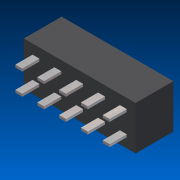
# Autodesk Inventor part: MOLEX
Saved by Autodesk Inventor 2015 SP1 (Build 190203100, 203)
## iProperties
Created: 2015-12-01
Part Number: MOLEX
Material: Generic
Document SubType Name: Modeling
Designer: User
Density: 1 g/cm^3
Appearance: Default
Author: User
Autodesk Inventor part; units mm, degrees
ref_plane "YZ Plane" through (0, 0, 0) normal (1, 0, 0) x (0, 1, 0)
ref_plane "XZ Plane" through (0, 0, 0) normal (0, 1, 0) x (-1, 0, 0)
ref_plane "XY Plane" through (0, 0, 0) normal (0, 0, 1) x (1, 0, 0)
sketch "Эскиз1" plane through (0, 0, 0) normal (0, 1, 0) x (-1, 0, 0)
  line L0 (6.5, -2.54) -> (-6.5, -2.54)
  line L1 (-6.5, -2.54) -> (-6.5, 2.54)
  line L2 (-6.5, 2.54) -> (6.5, 2.54)
  line L3 (6.5, 2.54) -> (6.5, -2.54)
  line L4 (0, -3.556) -> (0, 3.556) projected
  line L5 (9.1, 0) -> (-9.1, 0) projected
  point P0 (0, 0)
  dimension "d0" = 13
  dimension "d1" = 5.08
  constraints: 8 end point, 2 parallel, 1 horizontal, 1 perpendicular, 2 other
  measures "d0" distance of L1.end L2.end
  measures "d1" distance of L0.end L1.end
extrude "Выдавливание1" add sketch "Эскиз1" along normal blind 4.4
sketch "Эскиз2" plane through (0, 4.4, 0) normal (0, 1, 0) x (1, 0, 0)
  line L0 (-5.48, 1.67) -> (-4.68, 1.67)
  line L1 (-4.68, 1.67) -> (-4.68, 0.87)
  line L2 (-4.68, 0.87) -> (-5.48, 0.87)
  line L3 (-5.48, 0.87) -> (-5.48, 1.67)
  line L4 (-2.94, 1.67) -> (-2.14, 1.67)
  line L5 (-2.14, 1.67) -> (-2.14, 0.87)
  line L6 (-2.14, 0.87) -> (-2.94, 0.87)
  line L7 (-2.94, 0.87) -> (-2.94, 1.67)
  line L8 (-0.4, 1.67) -> (0.4, 1.67)
  line L9 (0.4, 1.67) -> (0.4, 0.87)
  line L10 (0.4, 0.87) -> (-0.4, 0.87)
  line L11 (-0.4, 0.87) -> (-0.4, 1.67)
  line L12 (2.14, 1.67) -> (2.94, 1.67)
  line L13 (2.94, 1.67) -> (2.94, 0.87)
  line L14 (2.94, 0.87) -> (2.14, 0.87)
  line L15 (2.14, 0.87) -> (2.14, 1.67)
  line L16 (4.68, 1.67) -> (5.48, 1.67)
  line L17 (5.48, 1.67) -> (5.48, 0.87)
  line L18 (5.48, 0.87) -> (4.68, 0.87)
  line L19 (4.68, 0.87) -> (4.68, 1.67)
  line L20 (-5.48, -0.87) -> (-4.68, -0.87)
  line L21 (-4.68, -0.87) -> (-4.68, -1.67)
  line L22 (-4.68, -1.67) -> (-5.48, -1.67)
  line L23 (-5.48, -1.67) -> (-5.48, -0.87)
  line L24 (-2.94, -0.87) -> (-2.14, -0.87)
  line L25 (-2.14, -0.87) -> (-2.14, -1.67)
  line L26 (-2.14, -1.67) -> (-2.94, -1.67)
  line L27 (-2.94, -1.67) -> (-2.94, -0.87)
  line L28 (-0.4, -0.87) -> (0.4, -0.87)
  line L29 (0.4, -0.87) -> (0.4, -1.67)
  line L30 (0.4, -1.67) -> (-0.4, -1.67)
  line L31 (-0.4, -1.67) -> (-0.4, -0.87)
  line L32 (2.14, -0.87) -> (2.94, -0.87)
  line L33 (2.94, -0.87) -> (2.94, -1.67)
  line L34 (2.94, -1.67) -> (2.14, -1.67)
  line L35 (2.14, -1.67) -> (2.14, -0.87)
  line L36 (4.68, -0.87) -> (5.48, -0.87)
  line L37 (5.48, -0.87) -> (5.48, -1.67)
  line L38 (5.48, -1.67) -> (4.68, -1.67)
  line L39 (4.68, -1.67) -> (4.68, -0.87)
  line L40 (0, 3.556) -> (0, -3.556) projected
  line L41 (-9.1, 0) -> (9.1, 0) projected
  point P0 (0, 0)
  dimension "d4" = 0.8
  dimension "d5" = 0.8
  dimension "d8" = 2.54
  dimension "d11" = 2.54
  constraints: 80 end point, 2 collinear, 2 horizontal, 2 parallel, 1 perpendicular, 1 vertical, 72 other
  measures "d4" distance of L1.end L2.end
  measures "d5" distance of L0.end L1.end
  measures "d8" distance of L0.start L4.start
  measures "d11" distance of L0.start L20.start
extrude "Выдавливание2" cut sketch "Эскиз2" against normal blind 4
sketch "Эскиз3" plane through (0, 0, 0) normal (0, -1, 0) x (1, 0, 0)
  line L0 (0, -3.556) -> (0, 3.556) projected
  line L1 (-9.1, 0) -> (9.1, 0) projected
  line L2 (-5.48, 1.42) -> (-4.68, 1.42)
  line L3 (-4.68, 1.42) -> (-4.68, 1.12)
  line L4 (-4.68, 1.12) -> (-5.48, 1.12)
  line L5 (-5.48, 1.12) -> (-5.48, 1.42)
  line L6 (-2.94, 1.42) -> (-2.14, 1.42)
  line L7 (-2.14, 1.42) -> (-2.14, 1.12)
  line L8 (-2.14, 1.12) -> (-2.94, 1.12)
  line L9 (-2.94, 1.12) -> (-2.94, 1.42)
  line L10 (-0.4, 1.42) -> (0.4, 1.42)
  line L11 (0.4, 1.42) -> (0.4, 1.12)
  line L12 (0.4, 1.12) -> (-0.4, 1.12)
  line L13 (-0.4, 1.12) -> (-0.4, 1.42)
  line L14 (2.14, 1.42) -> (2.94, 1.42)
  line L15 (2.94, 1.42) -> (2.94, 1.12)
  line L16 (2.94, 1.12) -> (2.14, 1.12)
  line L17 (2.14, 1.12) -> (2.14, 1.42)
  line L18 (4.68, 1.42) -> (5.48, 1.42)
  line L19 (5.48, 1.42) -> (5.48, 1.12)
  line L20 (5.48, 1.12) -> (4.68, 1.12)
  line L21 (4.68, 1.12) -> (4.68, 1.42)
  line L22 (-5.48, -1.12) -> (-4.68, -1.12)
  line L23 (-4.68, -1.12) -> (-4.68, -1.42)
  line L24 (-4.68, -1.42) -> (-5.48, -1.42)
  line L25 (-5.48, -1.42) -> (-5.48, -1.12)
  line L26 (-2.94, -1.12) -> (-2.14, -1.12)
  line L27 (-2.14, -1.12) -> (-2.14, -1.42)
  line L28 (-2.14, -1.42) -> (-2.94, -1.42)
  line L29 (-2.94, -1.42) -> (-2.94, -1.12)
  line L30 (-0.4, -1.12) -> (0.4, -1.12)
  line L31 (0.4, -1.12) -> (0.4, -1.42)
  line L32 (0.4, -1.42) -> (-0.4, -1.42)
  line L33 (-0.4, -1.42) -> (-0.4, -1.12)
  line L34 (2.14, -1.12) -> (2.94, -1.12)
  line L35 (2.94, -1.12) -> (2.94, -1.42)
  line L36 (2.94, -1.42) -> (2.14, -1.42)
  line L37 (2.14, -1.42) -> (2.14, -1.12)
  line L38 (4.68, -1.12) -> (5.48, -1.12)
  line L39 (5.48, -1.12) -> (5.48, -1.42)
  line L40 (5.48, -1.42) -> (4.68, -1.42)
  line L41 (4.68, -1.42) -> (4.68, -1.12)
  point P0 (0, 0)
  dimension "d16" = 0.8
  dimension "d17" = 0.3
  dimension "d20" = 2.54
  dimension "d23" = 2.54
  constraints: 80 end point, 2 collinear, 2 horizontal, 2 parallel, 1 perpendicular, 1 vertical, 72 other
  measures "d16" distance of L3.end L4.end
  measures "d17" distance of L2.end L3.end
  measures "d20" distance of L2.start L6.start
  measures "d23" distance of L2.start L22.start
extrude "Выдавливание3" add sketch "Эскиз3" along normal blind 2
